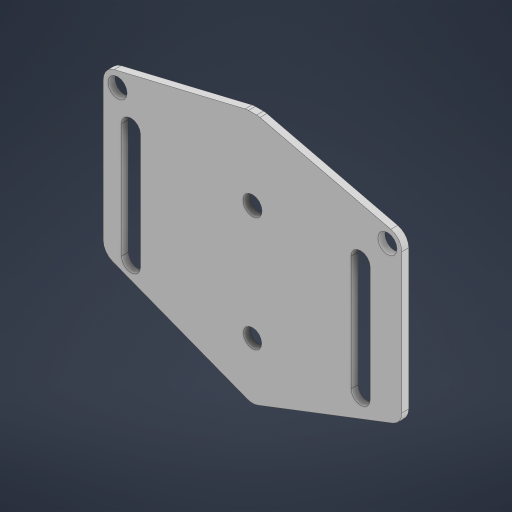
# Autodesk Inventor part: Part23
Saved by Autodesk Inventor 2023.2 (Build 272271000, 271)
## iProperties
Created: 2023-03-19
Part Number: Part23
Material: Generic
Document SubType Name: Modeling
Designer: Liam
Density: 1 g/cm^3
Appearance: Default
Author: Liam
Autodesk Inventor part; units mm, degrees
ref_plane "YZ Plane" through (0, 0, 0) normal (1, 0, 0) x (0, 1, 0)
ref_plane "XZ Plane" through (0, 0, 0) normal (0, 1, 0) x (-1, 0, 0)
ref_plane "XY Plane" through (0, 0, 0) normal (0, 0, 1) x (1, 0, 0)
sketch "Sketch1" plane through (0, 0, 0) normal (0, 0, 1) x (1, 0, 0)
  circle A0 centre (0, 0) radius 2.032 projected
  circle A1 centre (0, 25.4) radius 2.1082
  line L0 (26.0246, 26.6073) -> (26.0246, 1.2073)
  line L1 (21.8082, 26.6073) -> (21.8082, 1.2073)
  arc A2 (26.0246, 26.6073) -> (21.8082, 26.6073) centre (23.9164, 26.6073) ccw
  arc A3 (21.8082, 1.2073) -> (26.0246, 1.2073) centre (23.9164, 1.2073) ccw
  line L2 (-33.02, 2.1806) -> (-33.02, 33.0568)
  line L3 (33.02, 2.1806) -> (33.02, 33.0568)
  line L4 (0, 43.18) -> (0.8943, 43.18)
  line L5 (0, 43.18) -> (-0.8943, 43.18)
  line L6 (1.6353, 43.0923) -> (30.586, 36.1442)
  line L7 (-1.6353, 43.0923) -> (-30.586, 36.1442)
  line L8 (0, 0) -> (0, -12.7)
  line L9 (-30.9848, -0.7828) -> (-1.1398, -12.2616)
  line L10 (30.9848, -0.7828) -> (1.1398, -12.2616)
  arc A4 (-30.586, 36.1442) -> (-33.02, 33.0568) centre (-29.845, 33.0568) ccw
  arc A5 (-0.8943, 43.18) -> (-1.6353, 43.0923) centre (-0.8943, 40.005) ccw
  arc A6 (1.6353, 43.0923) -> (0.8943, 43.18) centre (0.8943, 40.005) ccw
  arc A7 (33.02, 33.0568) -> (30.586, 36.1442) centre (29.845, 33.0568) ccw
  arc A8 (30.9848, -0.7828) -> (33.02, 2.1806) centre (29.845, 2.1806) ccw
  arc A9 (-1.1398, -12.2616) -> (1.1398, -12.2616) centre (0, -9.2983) ccw
  arc A10 (-33.02, 2.1806) -> (-30.9848, -0.7828) centre (-29.845, 2.1806) ccw
  line L11 (-24.7754, 26.6073) -> (-24.7754, 1.2073)
  line L12 (-28.9918, 26.6073) -> (-28.9918, 1.2073)
  arc A11 (-24.7754, 26.6073) -> (-28.9918, 26.6073) centre (-26.8836, 26.6073) ccw
  arc A12 (-28.9918, 1.2073) -> (-24.7754, 1.2073) centre (-26.8836, 1.2073) ccw
  circle A13 centre (-29.845, 33.0568) radius 2.1082
  circle A14 centre (29.845, 33.0568) radius 2.1082
  point P0 (0, 0)
  point P1 (-33.02, 0)
  point P2 (33.02, 0)
  point P3 (-33.02, 35.56)
  point P4 (1.27, 43.18)
  point P5 (-1.27, 43.18)
  dimension "d1" = 4.2164
  dimension "d10" = 33.02
  dimension "d11" = 33.02
  dimension "d12" = 43.18
  dimension "d13" = 35.56
  dimension "d14" = 1.27
  dimension "d15" = 1.27
  dimension "d16" = 12.7
  dimension "d17" = 3.175
  dimension "d37" = 2.1082
  dimension "d38" = 25.4
  dimension "d39" = 4.2164
  dimension "d41" = 2.1082
  dimension "d43" = 4.2164
  dimension "d44" = 4.2164
  dimension "d45" = 4.2164
  constraints: 26 end point, 22 point on circle, 18 tangent, 14 centre point, 12 point on line, 6 equal radius, 3 vertical, 2 coincident, 2 horizontal, 4 other
  measures "d1" diameter of A1
  measures "d10" distance of L8.start point (-33.02, 0)
  measures "d11" distance of L8.start point (33.02, 0)
  measures "d12" distance of L8.start L4.start
  measures "d13" distance of point (-33.02, 0) point (-33.02, 35.56)
  measures "d14" distance of L4.start point (1.27, 43.18)
  measures "d15" distance of L4.start point (-1.27, 43.18)
  measures "d16" distance of L8.start L8.end
  measures "d17" radius of A4
  measures "d37" radius of A11
  measures "d38" distance of L11.start L11.end
  measures "d39" distance between parallel lines of L11 L12
  measures "d41" radius of A12
  measures "d43" distance between parallel lines of L1 L0
  measures "d44" diameter of A13
  measures "d45" diameter of A14
extrude "Extrusion3" add sketch "Sketch1" along normal blind 1.524
equation "\"d1\" = d43"
equation "\"d39\" = 2 * d37"
equation "\"d41\" = d37"
equation "\"d43\" = d39"
body "Solid2"
